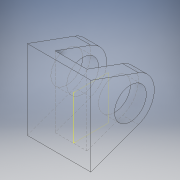
# Autodesk Inventor part: stick
Saved by Autodesk Inventor 2018 (Build 220112000, 112)
## iProperties
Created: 2018-01-21
Part Number: stick
Material: Generic
Document SubType Name: Modeling
Designer: omara
Density: 1 g/cm^3
Appearance: Default
Author: omara
Autodesk Inventor part; units mm, degrees
ref_plane "YZ Plane" through (0, 0, 0) normal (1, 0, 0) x (0, 1, 0)
ref_plane "XZ Plane" through (0, 0, 0) normal (0, 1, 0) x (-1, 0, 0)
ref_plane "XY Plane" through (0, 0, 0) normal (0, 0, 1) x (1, 0, 0)
sketch "Sketch1" plane through (0, 0, 0) normal (1, 0, 0) x (0, 1, 0)
  line L0 (0, 50) -> (0, -50)
  line L1 (0, -50) -> (59.9203, -28.1908)
  line L2 (0, 50) -> (59.9203, 28.1908)
  circle A0 centre (49.6597, 0) radius 20
  arc A1 (59.9203, -28.1908) -> (59.9203, 28.1908) centre (49.6597, 0) ccw
  point P0 (0, 0)
  dimension "d0" = 100
  dimension "d1" = 50
  dimension "d2" = 40
  dimension "d3" = 60
  dimension "d5" = 70
  dimension "d6" = 70
  constraints: 6 end point, 2 centre point, 2 point on circle, 2 tangent, 1 coincident, 1 vertical
  measures "d0" distance of L0.start L0.end
  measures "d1" distance of point (0, 0) L0.end
  measures "d2" diameter of A0
  measures "d3" diameter of A1
  measures "d5" angle of L0 L1
  measures "d6" angle of L0 L2
extrude "Extrusion1" add sketch "Sketch1" against normal blind 80
ref_plane "Work Plane1" through (-20, 0, 0) normal (1, 0, 0) x (0, 0, -1)
sketch "Sketch2" plane through (-20, 0, 0) normal (1, 0, 0) x (0, 0, -1)
  line L0 (-50, 0) -> (-28.1908, 59.9203) projected
  line L1 (50, 0) -> (-50, 0) projected
  line L2 (-50, 0) -> (50, 0)
  arc A0 (28.1908, 59.9203) -> (-28.1908, 59.9203) centre (0, 49.6597) ccw projected
  line L3 (-57.2418, 112.7643) -> (51.1454, 112.7643)
  line L4 (51.1454, 112.7643) -> (51.1454, 15.0485)
  line L5 (51.1454, 15.0485) -> (-57.2418, 15.0485)
  line L6 (-57.2418, 15.0485) -> (-57.2418, 112.7643)
  point P0 (0, 0)
  constraints: 10 end point, 2 horizontal, 2 parallel, 1 perpendicular
extrude "Extrusion2" cut sketch "Sketch2" against normal blind 40
body "Solid1"
